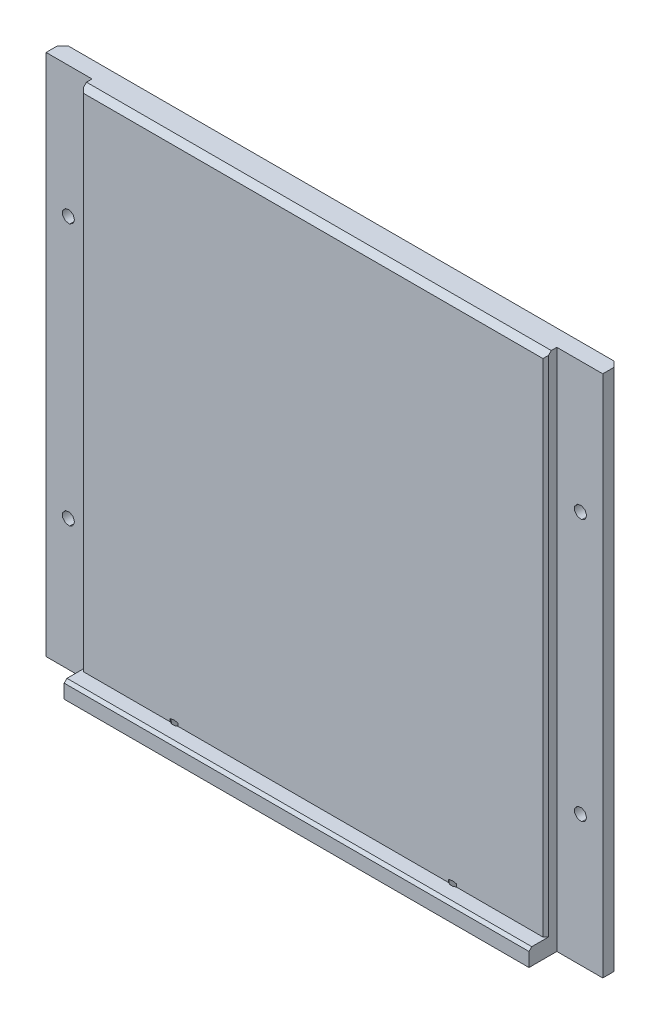
# Autodesk Inventor part: FrontPanel
Saved by Autodesk Inventor 2023 (Build 270158000, 158)
## iProperties
Created: 2022-08-05
Part Number: FrontPanel
Material: Aluminum 6061
Document SubType Name: Modeling
Designer: Aditya Bansal
Density: 2.7 g/cm^3
Appearance: Aluminum - Flat
Mass: 119.819 g
Surface Area: 210.46 cm^2
Volume: 44.3775 cm^3
Author: Aditya Bansal
Autodesk Inventor part; units mm, degrees
ref_plane "YZ Plane" through (0, 0, 0) normal (1, 0, 0) x (0, 1, 0)
ref_plane "XZ Plane" through (0, 0, 0) normal (0, 1, 0) x (-1, 0, 0)
ref_plane "XY Plane" through (0, 0, 0) normal (0, 0, 1) x (1, 0, 0)
sketch "Sketch1" plane through (0, 0, 0) normal (0, 0, 1) x (1, 0, 0)
  line L0 (0, 0) -> (100, 0)
  line L1 (100, 0) -> (100, 94)
  line L2 (100, 94) -> (0, 94)
  line L3 (0, 94) -> (0, 0)
  dimension "d0" = 100
  dimension "d1" = 94
  constraints: 8 end point, 2 parallel, 1 horizontal, 1 perpendicular
  measures "d0" distance of L1.end L2.end
  measures "d1" distance of L0.end L1.end
extrude "Extrusion1" add sketch "Sketch1" along normal blind 3
sketch "Sketch2" plane through (0, 0, 3) normal (0, 0, 1) x (1, 0, 0)
  line L0 (100, 94) -> (0, 94) projected
  line L1 (8.25, 94) -> (91.75, 94)
  line L2 (91.75, 94) -> (91.75, 0)
  line L3 (91.75, 0) -> (8.25, 0)
  line L4 (8.25, 0) -> (8.25, 94)
  line L5 (100, 0) -> (100, 94) construction
  line L6 (100, 94) -> (92, 94) construction
  line L7 (92, 94) -> (92, 0) construction
  line L8 (92, 0) -> (100, 0) construction
  line L9 (100, 0) -> (100, 94) construction
  line L10 (0, 94) -> (8, 94) construction
  line L11 (8, 94) -> (8, 0) construction
  line L12 (8, 0) -> (0, 0) construction
  line L13 (0, 0) -> (0, 94) construction
  line L14 (0, 0) -> (100, 0) construction
  dimension "d4" = 8
  dimension "d5" = 0.25
  dimension "d6" = 0.25
  constraints: 24 end point, 6 parallel, 3 horizontal, 3 perpendicular, 2 collinear, 2 point on line
  measures "d4" distance of L0.end L10.end
  measures "d5" distance between parallel lines of L4 L11
  measures "d6" distance between parallel lines of L7 L2
extrude "Extrusion2" add sketch "Sketch2" along normal blind 2
sketch "Sketch4" plane through (0, 0, 0) normal (0, -1, 0) x (1, 0, 0)
  line L0 (91.75, 5) -> (8.25, 5) projected
  line L1 (8.25, 5) -> (91.75, 5)
  line L2 (91.75, 5) -> (91.75, 8)
  line L3 (91.75, 8) -> (8.25, 8)
  line L4 (8.25, 8) -> (8.25, 5)
  line L5 (91.75, 3) -> (91.75, 5) projected
  line L6 (0, 0) -> (100, 0) projected
  dimension "d10" = 8
  constraints: 8 end point, 2 parallel, 1 collinear, 1 horizontal, 1 perpendicular
  measures "d10" distance between parallel lines of L3 L6
extrude "Extrusion3" add sketch "Sketch4" against normal blind 3
sketch "Sketch6" plane through (0, 0, 0) normal (0, -1, 0) x (1, 0, 0)
  line L0 (0, 0) -> (100, 0) projected
  line L1 (91.75, 8) -> (8.25, 8) projected
  line L2 (100, 0) -> (100, 3) projected
  point P0 (25, 4)
  point P1 (75, 4)
  dimension "d20" = 8
  dimension "d21" = 4
  dimension "d22" = 100
  dimension "d23" = 25
  dimension "d24" = 50
  constraints: 1 horizontal alignment
  measures "d20" distance between parallel lines of L0 L1
  measures "d21" distance from line of L0 point (25, 4)
  measures "d22" distance of L0.start L0.end
  measures "d23" distance from line of L2 point (75, 4)
  measures "d24" distance of point (75, 4) point (25, 4)
hole "Hole1" at (25, 0, 4) at (75, 0, 4) direction (0, 1, 0) diameter 2.459 depth 3.5 tip angle 118 thread size "M3x0.5" class "6H" standard "ANSI Metric M Profile"
sketch "Sketch7" plane through (0, 0, 0) normal (0, 0, -1) x (-1, 0, 0)
  line L0 (-91.75, 94) -> (-91.75, 0) projected
  line L1 (-8.25, 0) -> (-8.25, 94) projected
  line L2 (-100, 0) -> (-100, 94) projected
  line L3 (0, 94) -> (0, 0) projected
  line L4 (-100, 94) -> (0, 94) projected
  point P0 (-96, 70.5)
  point P1 (-4, 70.5)
  point P2 (-96, 23.5)
  point P3 (-4, 23.5)
  dimension "d32" = 8.25
  dimension "d33" = 4
  dimension "d34" = 4
  dimension "d35" = 94
  dimension "d36" = 23.5
  dimension "d39" = 47
  constraints: 1 horizontal alignment, 1 vertical, 2 other
  measures "d32" distance between parallel lines of L0 L2
  measures "d33" distance from line of point (-96, 70.5) L2
  measures "d34" distance from line of L3 point (-4, 70.5)
  measures "d35" distance of L3.start L3.end
  measures "d36" distance from line of L4 point (-4, 70.5)
  measures "d39" distance of point (-96, 70.5) point (-96, 23.5)
hole "Hole2" at (96, 70.5, 0) at (4, 70.5, 0) at (96, 23.5, 0) at (4, 23.5, 0) direction (0, 0, 1) diameter 2.2 depth 3.5 tip angle 118 countersink diameter 4.4 countersink angle 90 clearance for "Flat Head Machine Screw" size "M2" standard "Ansi Metric M Profile"
chamfer "Chamfer2" distance 0.5 angle 45 3 edges at (8.25, 48.5, 5) (91.75, 48.5, 5) (50, 3, 8)
chamfer "Chamfer3" distance 1 angle 45 1 edges at (50, 94, 5)
chamfer "Chamfer4" distance 1 angle 45 2 edges at (0, 47, 0) (100, 47, 0)
equation "\"d6\" = d5"
equation "\"d21\" = 0.5 * d20"
equation "\"d23\" = 0.25 * d22"
equation "\"d24\" = 2 * d23"
equation "\"d34\" = d33"
equation "\"d36\" = 0.25 * d35"
equation "\"d39\" = 2 * d36"
body "Solid1"
